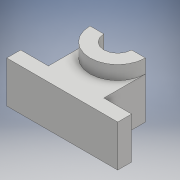
# Autodesk Inventor part: 1
Saved by Autodesk Inventor 2017 (Build 210142000, 142)
## iProperties
Part Number: 1
Material: 一般
Document SubType Name: Modeling
Designer: Brian
Mass: 60 g
Surface Area: 123.708 cm^2
Volume: 60 cm^3
Density: 1 g/cm^3
Appearance: 預設
Author: Brian
Autodesk Inventor part; units mm, degrees
ref_plane "YZ Plane" through (0, 0, 0) normal (1, 0, 0) x (0, 1, 0)
ref_plane "XZ Plane" through (0, 0, 0) normal (0, 1, 0) x (-1, 0, 0)
ref_plane "XY Plane" through (0, 0, 0) normal (0, 0, 1) x (1, 0, 0)
sketch "草圖1" plane through (0, 0, 0) normal (0, 0, 1) x (1, 0, 0)
  line L0 (0, 0) -> (80, 0)
  line L1 (80, 0) -> (80, 10)
  line L2 (80, 10) -> (0, 10)
  line L3 (0, 10) -> (0, 0)
  dimension "d0" = 80
  dimension "d1" = 10
  constraints: 8 end point, 2 parallel, 1 horizontal, 1 perpendicular
  measures "d0" distance of L0.start L0.end
  measures "d1" distance of L2.end L0.start
extrude "擠出1" add sketch "草圖1" along normal blind 30
sketch "草圖2" plane through (0, 0, 30) normal (0, 0, 1) x (1, 0, 0)
  line L0 (80, 10) -> (0, 10) projected
  line L1 (20, 10) -> (60, 10)
  line L2 (60, 10) -> (60, 40)
  line L3 (60, 40) -> (20, 40)
  line L4 (20, 40) -> (20, 10)
  point P0 (0, 0)
  dimension "d4" = 20
  dimension "d5" = 20
  dimension "d6" = 30
  constraints: 8 end point, 2 parallel, 1 horizontal, 1 perpendicular, 1 point on line
  measures "d4" distance from line of L0.end L4
  measures "d5" distance from line of L0.start L2
  measures "d6" distance of L1.end L2.end
extrude "擠出2" add sketch "草圖2" against normal up to surface (30 mm away)
sketch "草圖3" plane through (0, 0, 30) normal (0, 0, 1) x (1, 0, 0)
  line L0 (60, 40) -> (20, 40) projected
  circle A0 centre (40, 40) radius 10
  point P0 (0, 0)
  dimension "d9" = 20
  constraints: 1 centre point, 1 midpoint
  measures "d9" diameter of A0
extrude "擠出3" cut sketch "草圖3" against normal blind 30
sketch "草圖4" plane through (0, 0, 30) normal (0, 0, 1) x (1, 0, 0)
  arc A0 (30, 40) -> (50, 40) centre (40, 40) ccw projected
  line L0 (30, 40) -> (20, 40) projected
  circle A1 centre (40, 40) radius 20
  circle A2 centre (40, 40) radius 10
  line L1 (20, 40) -> (30, 40)
  line L2 (60, 40) -> (50, 40) projected
  line L3 (50, 40) -> (60, 40)
  line L4 (60, 10) -> (60, 40) projected
  point P0 (0, 0)
  constraints: 4 end point, 2 coincident, 2 point on circle, 1 centre point, 1 collinear, 1 horizontal alignment, 1 point on line, 2 other
extrude "擠出4" add sketch "草圖4" along normal blind 10 contours A0 L2 A1 L0
